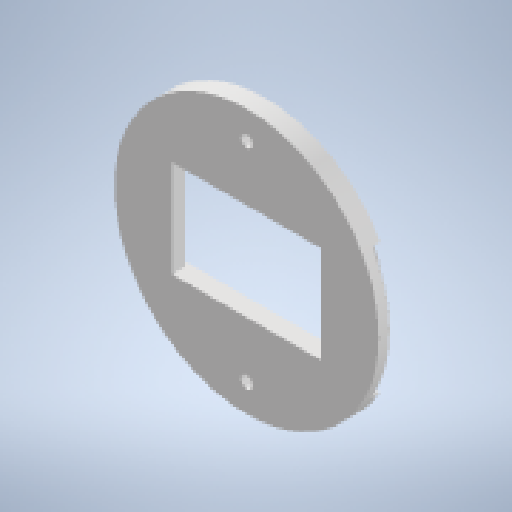
# Autodesk Inventor part: FilmGuide
Saved by Autodesk Inventor 2023 (Build 270158000, 158)
## iProperties
Created: 2022-10-31
Part Number: FilmGuide
Material: Generic
Document SubType Name: Modeling
Designer: Piotr
Density: 1 g/cm^3
Appearance: Default
Author: Piotr
Autodesk Inventor part; units mm, degrees
ref_plane "YZ Plane" through (0, 0, 0) normal (1, 0, 0) x (0, 1, 0)
ref_plane "XZ Plane" through (0, 0, 0) normal (0, 1, 0) x (-1, 0, 0)
ref_plane "XY Plane" through (0, 0, 0) normal (0, 0, 1) x (1, 0, 0)
sketch "Sketch1" plane through (0, 0, 0) normal (0, 0, 1) x (1, 0, 0)
  circle A0 centre (0, 28) radius 1.6 projected
  circle A1 centre (0, -28) radius 1.6 projected
  arc A2 (-32.9803, -13) -> (32.9803, -13) centre (0, 0) ccw projected
  arc A3 (32.9803, -13) -> (32.9803, 13) centre (0, 0) ccw projected
  arc A4 (32.9803, 13) -> (-32.9803, 13) centre (0, 0) ccw projected
  arc A5 (-32.9803, 13) -> (-32.9803, -13) centre (0, 0) ccw projected
extrude "Extrusion1" add sketch "Sketch1" along normal blind 5
sketch "Sketch2" plane through (0, 0, 0) normal (0, 0, -1) x (-1, 0, 0)
  line L0 (-35.45, 17.5) -> (35.45, 17.5)
  line L1 (35.45, 17.5) -> (35.45, -17.5)
  line L2 (35.45, -17.5) -> (-35.45, -17.5)
  line L3 (-35.45, -17.5) -> (-35.45, 17.5)
  line L4 (-35.45, 17.5) -> (35.45, -17.5) construction
  line L5 (35.45, 17.5) -> (-35.45, -17.5) construction
  circle A0 centre (0, 0) radius 35.45 projected
  point P0 (-30.8294, 17.5)
  point P1 (-30.8294, -17.5)
  point P2 (30.8294, -17.5)
  point P3 (30.8294, 17.5)
  dimension "d2" = 35
  constraints: 12 end point, 2 midpoint, 2 parallel, 1 horizontal, 1 perpendicular, 1 tangent
  measures "d2" distance between parallel lines of L2 L0
extrude "Extrusion2" cut sketch "Sketch2" against normal blind 0.2 contours L0 A0 L2
sketch "Sketch3" plane through (0, 0, 0.2) normal (0, 0, -1) x (-1, 0, 0)
  line L0 (-20, -13) -> (-20, 13) projected
  line L1 (-20, 13) -> (20, 13) projected
  line L2 (20, 13) -> (20, -13) projected
  line L3 (20, -13) -> (-20, -13) projected
  circle A0 centre (0, 28) radius 1.6 projected
  circle A1 centre (0, -28) radius 1.6 projected
  circle A2 centre (0, 0) radius 34.25 projected
extrude "Extrusion3" cut sketch "Sketch3" against normal through all contours L0 L1 L2 L3
chamfer "Chamfer1" distance 2 angle 45 2 edges at (-35.45, 0, 0.2) (35.3622, -2.4938, 0.2)
sketch "Sketch4" plane through (0, 0, 0.2) normal (0, 0, -1) x (-1, 0, 0)
  line L0 (-20, 13) -> (20, 13) projected
  line L1 (20, -13) -> (-20, -13) projected
  line L2 (-20, -13) -> (-20, 13) projected
  line L3 (20, 13) -> (20, -13) projected
  circle A0 centre (0, 0) radius 35.45 projected
  line L4 (20, 13) -> (-20, 13) projected
  line L5 (-20, 13) -> (-32.9803, 13)
  line L6 (-20, 13) -> (-20, -13) projected
  line L7 (-20, -13) -> (-32.9803, -13)
  arc A1 (-30.8294, 17.5) -> (-30.8294, -17.5) centre (0, 0) ccw projected
  line L8 (-20, -13) -> (20, -13) projected
  line L9 (20, -13) -> (32.9803, -13)
  circle A2 centre (0, 0) radius 35.45 projected
  line L10 (20, -13) -> (20, 13) projected
  line L11 (20, 13) -> (32.9803, 13)
  point P0 (26.4902, -13)
  constraints: 8 end point, 4 point on circle, 2 point on line, 1 collinear, 1 horizontal, 1 midpoint
extrude "Extrusion4" cut sketch "Sketch4" against normal blind 1.3 contours L2 L7 A0 L5 | L11 A0 L9 L3
body "Solid1"
